Autodesk Inventor part; units mm, degrees
(part 2 of 2)
sketch "Sketch182" plane through (0, 0, 82.74) normal (0, 0, 1) x (1, 0, 0)
  circle A0 centre (-26.5, 130) radius 1.5
  line L0 (-22.5, 136) -> (-22.5, 124) projected
  line L1 (-30.5, 124) -> (-30.5, 136) projected
  line L2 (-22.5, 124) -> (-30.5, 124) projected
  line L3 (-30.5, 136) -> (-22.5, 136) projected
  point P0 (0, 0)
  dimension "d607" = 8
  dimension "d608" = 4
  dimension "d609" = 12
  dimension "d610" = 6
  dimension "d611" = 3
  constraints: 1 centre point
  measures "d607" distance between parallel lines of L0 L1
  measures "d608" distance from line of L0 A0.centre
  measures "d609" distance between parallel lines of L2 L3
  measures "d610" distance from line of L3 A0.centre
  measures "d611" diameter of A0
extrude "Extrusion120" cut sketch "Sketch182" against normal blind 6 contours A0
ref_plane "Work Plane22" through (0, 0, 77) normal (0, 0, 1) x (1, 0, 0)
sketch "Sketch192" plane through (0, 55, 150) normal (0, 1, 0) x (1, 0, 0)
  line L0 (62, 25) -> (57, 25)
  line L1 (57, 25) -> (57, 30)
  line L2 (57, 30) -> (62, 30)
  line L3 (62, 30) -> (62, 25)
  line L4 (62, 25) -> (12, 25) projected
  line L5 (62, 75) -> (62, 25) projected
  line L6 (62, 75) -> (57, 75)
  line L7 (57, 75) -> (57, 70)
  line L8 (57, 70) -> (62, 70)
  line L9 (62, 70) -> (62, 75)
  line L10 (12, 25) -> (17, 25)
  line L11 (17, 25) -> (17, 30)
  line L12 (17, 30) -> (12, 30)
  line L13 (12, 30) -> (12, 25)
  line L14 (12, 75) -> (17, 75)
  line L15 (17, 75) -> (17, 70)
  line L16 (17, 70) -> (12, 70)
  line L17 (12, 70) -> (12, 75)
  point P0 (0, 150)
  dimension "d635" = 5
  constraints: 32 end point, 8 parallel, 7 equal length, 4 horizontal, 4 perpendicular, 3 point on line, 1 coincident
  measures "d635" distance of L1.end L2.end
extrude "Extrusion122" add sketch "Sketch192" against normal blind 3
sketch "Sketch193" plane through (-5, -5, 150) normal (0, -1, 0) x (1, 0, 0)
  line L0 (86.0111, 0) -> (16.0111, 0)
  line L1 (16.0111, 0) -> (16.0111, -137.496)
  line L2 (16.0111, -137.496) -> (86.0111, -137.496)
  line L3 (86.0111, -137.496) -> (86.0111, 0)
  line L4 (0, 0) -> (155, 0) projected
  line L5 (76.0111, -37.496) -> (76.0111, -87.496) projected
  line L6 (26.0111, -87.496) -> (26.0111, -37.496) projected
  line L7 (76.0111, -87.496) -> (26.0111, -87.496) projected
  point P0 (5, -150)
  dimension "d638" = 10
  dimension "d639" = 10
  dimension "d640" = 50
  constraints: 8 end point, 2 parallel, 1 horizontal, 1 perpendicular, 1 point on line
  measures "d638" distance between parallel lines of L3 L5
  measures "d639" distance between parallel lines of L1 L6
  measures "d640" distance between parallel lines of L7 L2
extrude "Extrusion123" add sketch "Sketch193" along normal blind 10
sketch "Sketch194" plane through (-5, -15, 150) normal (0, -1, 0) x (1, 0, 0)
  line L0 (76.0111, -37.496) -> (26.0111, -37.496) projected
  line L1 (76.0111, -87.496) -> (76.0111, -37.496) projected
  line L2 (26.0111, -37.496) -> (76.0111, -37.496)
  line L3 (76.0111, -37.496) -> (76.0111, -87.496)
  line L4 (76.0111, -87.496) -> (26.0111, -87.496)
  line L5 (26.0111, -87.496) -> (26.0111, -37.496)
  point P0 (5, -150)
  constraints: 8 end point, 2 parallel, 1 horizontal, 1 perpendicular
extrude "Extrusion124" cut sketch "Sketch194" against normal up to surface (15 mm away)
sketch "Sketch195" plane through (72, 0, 150) normal (0, 1, 0) x (1, 0, 0)
  line L0 (-0.9889, 87.496) -> (-0.9889, 37.496) projected
  line L1 (-0.9889, 37.496) -> (-5.9889, 37.496)
  line L2 (-5.9889, 37.496) -> (-5.9889, 42.496)
  line L3 (-5.9889, 42.496) -> (-0.9889, 42.496)
  line L4 (-0.9889, 42.496) -> (-0.9889, 37.496)
  line L5 (-50.9889, 87.496) -> (-0.9889, 87.496) projected
  line L6 (-0.9889, 87.496) -> (-5.9889, 87.496)
  line L7 (-5.9889, 87.496) -> (-5.9889, 82.496)
  line L8 (-5.9889, 82.496) -> (-0.9889, 82.496)
  line L9 (-0.9889, 82.496) -> (-0.9889, 87.496)
  line L10 (-50.9889, 37.496) -> (-50.9889, 87.496) projected
  line L11 (-50.9889, 87.496) -> (-45.9889, 87.496)
  line L12 (-45.9889, 87.496) -> (-45.9889, 82.496)
  line L13 (-45.9889, 82.496) -> (-50.9889, 82.496)
  line L14 (-50.9889, 82.496) -> (-50.9889, 87.496)
  line L15 (-0.9889, 37.496) -> (-50.9889, 37.496) projected
  line L16 (-50.9889, 37.496) -> (-45.9889, 37.496)
  line L17 (-45.9889, 37.496) -> (-45.9889, 42.496)
  line L18 (-45.9889, 42.496) -> (-50.9889, 42.496)
  line L19 (-50.9889, 42.496) -> (-50.9889, 37.496)
  point P0 (-72, 150)
  point P1 (-0.9889, 82.496)
  dimension "d645" = 5
  constraints: 32 end point, 8 parallel, 7 equal length, 4 horizontal, 4 perpendicular
  measures "d645" distance of L16.end L17.end
extrude "Extrusion125" add sketch "Sketch195" against normal blind 3 contours L0 L8 L7 L5 | L0 L1 L2 L3 | L12 L13 L10 L5 | L15 L10 L18 L17
sketch "Sketch196" plane through (-65, 65, 150) normal (0, -1, 0) x (1, 0, 0)
  line L0 (12, -83.999) -> (9, -83.999)
  line L1 (9, -83.999) -> (9, -153)
  line L2 (9, -153) -> (12, -153)
  line L3 (12, -153) -> (12, -83.999)
  line L4 (5, -86.999) -> (5, -175) projected
  line L5 (0, -86.999) -> (5, -86.999) projected
  line L6 (170, -150) -> (190, -150) projected
  line L7 (190, -150) -> (170, -150) projected
  line L8 (210, -150) -> (190, -150) projected
  line L9 (190, -150) -> (95, -150) projected
  line L10 (95, -150) -> (142, -150) projected
  line L11 (142, -150) -> (190, -150) projected
  line L12 (190, -150) -> (210, -150) projected
  line L13 (132.0208, -150) -> (128.4853, -150) projected
  line L14 (128.4853, -150) -> (107.9792, -150) projected
  line L15 (107.9792, -150) -> (111.5147, -150) projected
  line L16 (111.5147, -150) -> (132.0208, -150) projected
  line L17 (150, -150) -> (160, -150) projected
  line L18 (160, -150) -> (150, -150) projected
  line L19 (65, -155) -> (210, -155) projected
  line L20 (65, -155) -> (210, -155) projected
  line L21 (65, -155) -> (210, -155) projected
  point P0 (65, -150)
  point P1 (5, -150)
  dimension "d648" = 4
  dimension "d649" = 3
  dimension "d650" = 3
  dimension "d651" = 5
  dimension "d652" = 3
  constraints: 8 end point, 2 parallel, 1 horizontal, 1 perpendicular
  measures "d648" distance between parallel lines of L4 L1
  measures "d649" distance from line of point (5, -150) L2
  measures "d650" distance between parallel lines of L0 L5
  measures "d651" distance from line of L21 point (5, -150)
  measures "d652" distance between parallel lines of L1 L3
extrude "Extrusion126" cut sketch "Sketch196" against normal up to surface (120 mm away)
sketch "Sketch197" plane through (-60, 65, -5) normal (-1, 0, 0) x (0, 0, 1)
  line L0 (-18, 117) -> (3, 117)
  line L1 (3, 117) -> (3, 114)
  line L2 (3, 114) -> (-18, 114)
  line L3 (-18, 114) -> (-18, 117)
  line L4 (68.001, 120) -> (-20, 120) projected
  line L5 (-15, 120) -> (-15, 3) projected
  line L6 (0, 120) -> (0, 3) projected
  point P0 (5, -65)
  dimension "d655" = 3
  dimension "d656" = 3
  dimension "d657" = 3
  dimension "d658" = 3
  constraints: 8 end point, 2 parallel, 1 horizontal, 1 perpendicular
  measures "d655" distance between parallel lines of L4 L0
  measures "d656" distance of L0.end L1.end
  measures "d657" distance between parallel lines of L5 L3
  measures "d658" distance between parallel lines of L6 L1
extrude "Extrusion127" cut sketch "Sketch197" against normal up to surface (210 mm away) contours L0 L5 L2 L3 | L0 L6 L2 L5 | L0 L1 L2 L6
sketch "Sketch198" plane through (-5, -5, 150) normal (-1, 0, 0) x (0, 0, 1)
  line L0 (-173, 6) -> (-152, 6)
  line L1 (-152, 6) -> (-152, 3)
  line L2 (-152, 3) -> (-173, 3)
  line L3 (-173, 3) -> (-173, 6)
  line L4 (-175, 0) -> (0, 0) projected
  point P0 (-150, 5)
  point P1 (-155, 0)
  point P2 (-170, 0)
  dimension "d661" = 3
  dimension "d662" = 3
  dimension "d663" = 3
  dimension "d664" = 3
  constraints: 8 end point, 2 parallel, 1 horizontal, 1 perpendicular
  measures "d661" distance between parallel lines of L4 L2
  measures "d662" distance between parallel lines of L0 L2
  measures "d663" distance from line of point (-155, 0) L1
  measures "d664" distance from line of L3 point (-170, 0)
extrude "Extrusion128" cut sketch "Sketch198" against normal up to surface (155 mm away)
sketch "Sketch203" plane through (0, 0, 150) normal (0, 0, 1) x (1, 0, 0)
  line L0 (60, 28.3) -> (50, 28.3) projected
  line L1 (48.4237, 33.6572) -> (60, 33.6572)
  line L2 (60, 33.6572) -> (60, 28.3)
  line L3 (60, 28.3) -> (48.4237, 28.3)
  line L4 (48.4237, 28.3) -> (48.4237, 33.6572)
  point P0 (0, 0)
  point P1 (53, 28.3)
  point P2 (57, 28.3)
  constraints: 8 end point, 2 parallel, 1 horizontal, 1 perpendicular
extrude "Extrusion129" cut sketch "Sketch203" against normal up to surface (150 mm away)
sketch "Sketch205" plane through (0, 0, 67) normal (0, 0, 1) x (1, 0, 0)
  line L0 (0.6988, 151.5) -> (0.6988, 113) projected
  line L1 (-9.9078, 140) -> (-9.9078, 113) projected
  line L2 (-22.5, 124) -> (-30.5, 124) projected
  line L3 (-30.5, 136) -> (-22.5, 136) projected
  circle A0 centre (-4.6012, 130) radius 15.5
  circle A1 centre (-4.6012, 130) radius 17.2238
  point P0 (0, 0)
  dimension "d678" = 10.6066
  dimension "d679" = 12
  dimension "d680" = 31
  dimension "d681" = 6
  dimension "d683" = 5.3
  constraints: 2 centre point, 1 coincident
  measures "d678" distance between parallel lines of L0 L1
  measures "d679" distance between parallel lines of L2 L3
  measures "d680" diameter of A0
  measures "d681" distance from line of L3 A0.centre
  measures "d683" distance from line of L0 A0.centre
extrude "Extrusion130" add sketch "Sketch205" along normal blind 10 contours A1 L0 A0 | L0 A0 L1 A1 | L1 A0 L0 A1
sketch "Sketch206" plane through (0, 0, 67) normal (0, 0, 1) x (1, 0, 0)
  circle A0 centre (-4.6012, 130) radius 8.89
  arc A1 (0.6988, 144.5657) -> (-9.9078, 144.5633) centre (-4.6012, 130) ccw projected
  point P0 (0, 0)
  point P1 (5.2095, 118)
  point P2 (-14.4119, 118)
  dimension "d686" = 17.78
  constraints: 1 centre point, 1 concentric
  measures "d686" diameter of A0
extrude "Extrusion131" cut sketch "Sketch206" against normal up to surface (4 mm away)
sketch "Sketch207" plane through (0.6988, 140, 67) normal (-1, 0, 0) x (0, 0, 1)
  line L0 (31.7021, 6.386) -> (31.7021, 0)
  line L1 (31.7021, 0) -> (0, 0)
  line L2 (0, 0) -> (0, 4.5657) projected
  line L3 (0, 0) -> (0, 4.8278)
  line L4 (0, 4.8278) -> (10, 4.8278)
  line L5 (10, 6.386) -> (10, 7.2238) projected
  line L6 (10, 4.8278) -> (10, 6.386)
  line L7 (10, 6.386) -> (31.7021, 6.386)
  line L8 (0, 0) -> (36.0104, 0) projected
  point P0 (-67, -140)
  point P1 (10, 6.3881)
  constraints: 12 end point, 3 perpendicular, 2 point on line, 2 vertical, 1 parallel
extrude "Extrusion132" cut sketch "Sketch207" against normal blind 10
sketch "Sketch208" plane through (-8.14, 140, 67) normal (1, 0, 0) x (0, 0, -1)
  line L0 (0, 4) -> (0, 0) projected
  line L1 (0, 0) -> (-23.1716, 0) projected
  line L2 (0, 4) -> (-16.0959, 4)
  line L3 (-16.0959, 4) -> (-16.0959, 0)
  line L4 (-16.0959, 0) -> (0, 0)
  line L5 (0, 0) -> (0, 4)
  point P0 (67, -140)
  constraints: 8 end point, 2 parallel, 1 horizontal, 1 perpendicular, 1 point on line
extrude "Extrusion133" cut sketch "Sketch208" against normal blind 10
sketch "Sketch209" plane through (0, 0, 150) normal (0, 0, 1) x (1, 0, 0)
  line L0 (11.0111, -5) -> (11.0111, -15) projected
  line L1 (81.0111, -5) -> (81.0111, -15) projected
  line L2 (11.0111, -15) -> (81.0111, -15)
  line L3 (81.0111, -15) -> (81.0111, -10)
  line L4 (81.0111, -10) -> (11.0111, -10)
  line L5 (11.0111, -10) -> (11.0111, -15)
  point P0 (0, 0)
  dimension "d693" = 5
  dimension "d694" = 70
  constraints: 8 end point, 2 parallel, 1 horizontal, 1 midpoint, 1 perpendicular
  measures "d693" distance between parallel lines of L2 L4
  measures "d694" distance of L3.end L4.end
extrude "Extrusion134" cut sketch "Sketch209" against normal up to surface (137.496 mm away)
sketch "Sketch210" plane through (0, 0, 150) normal (0, 0, 1) x (1, 0, 0)
  line L0 (0, 27) -> (72, 27) projected
  line L1 (47.5453, 27) -> (62.1225, 27)
  line L2 (62.1225, 27) -> (62.1225, 32.383)
  line L3 (62.1225, 32.383) -> (47.5453, 32.383)
  line L4 (47.5453, 32.383) -> (47.5453, 27)
  point P0 (0, 0)
  constraints: 8 end point, 2 parallel, 1 horizontal, 1 perpendicular, 1 point on line
extrude "Extrusion135" cut sketch "Sketch210" against normal up to surface (150 mm away)
sketch "Sketch211" plane through (-9.9078, 151.5, 92.4038) normal (1, 0, 0) x (0, 0, -1)
  line L0 (25.4038, -6.9367) -> (25.4038, -7.5) projected
  line L1 (25.4038, -6.9367) -> (15.4038, -6.9367) projected
  line L2 (25.4038, -7.5) -> (15.4038, -7.5)
  line L3 (15.4038, -7.5) -> (15.4038, -6.9367)
  line L4 (15.4038, -6.9367) -> (25.4038, -6.9367)
  line L5 (25.4038, -6.9367) -> (25.4038, -7.5)
  point P0 (92.4038, -151.5)
  constraints: 8 end point, 2 parallel, 1 horizontal, 1 perpendicular
extrude "Extrusion136" cut sketch "Sketch211" against normal blind 25.4
thread "Thread9" size "5-40 UNC" class "2B" standard "ANSI Unified Screw Threads" full length
sketch "Sketch212" plane through (-35, 70, 150) normal (1, 0, 0) x (0, 0, -1)
  circle A0 centre (50, 60) radius 10 projected
  line L0 (83, 20) -> (83, 90) projected
  line L1 (150, 110) -> (150, 0) projected
  point P0 (150, -70)
  dimension "d703" = 33
  dimension "d704" = 100
  measures "d703" distance from line of L0 A0.centre
  measures "d704" distance from line of L1 A0.centre
ref_plane "Work Plane24" through (145, 62, -5) normal (0, 0, -1) x (-1, 0, 0)
sketch "Sketch213" plane through (-65, 65, 150) normal (-1, 0, 0) x (0, 0, 1)
  line L0 (-87, 115) -> (-150, 115) projected
  line L1 (-86.999, 120) -> (-86.999, 0) projected
  line L2 (-150, 5) -> (-150, 115) projected
  line L3 (-87, 5) -> (-150, 5) projected
  line L4 (-173, 117) -> (-152, 117) projected
  line L5 (-152, 114) -> (-173, 114) projected
  line L6 (-152, 117) -> (-152, 114) projected
  line L7 (-173, 114) -> (-173, 117) projected
  line L8 (-86.999, 120) -> (-175, 120) projected
  line L9 (-86.999, 120) -> (-175, 120)
  line L10 (-175, 120) -> (-175, 0)
  line L11 (-175, 0) -> (-86.999, 0)
  line L12 (-86.999, 0) -> (-86.999, 120)
  point P0 (-150, -65)
  point P1 (-86.999, 0)
  constraints: 8 end point, 2 parallel, 1 horizontal, 1 perpendicular
ref_plane "Work Plane25" through (-90.4, 65, 150) normal (-1, 0, 0) x (0, 0, 1)
sketch "Sketch214" plane through (-90.4, 65, 150) normal (-1, 0, 0) x (0, 0, 1)
  line L0 (-173, 117) -> (-152, 117) projected
  line L1 (-152, 114) -> (-173, 114) projected
  line L2 (-152, 117) -> (-152, 114) projected
  line L3 (-173, 114) -> (-173, 117) projected
  line L4 (-87, 115) -> (-150, 115) projected
  line L5 (-150, 5) -> (-150, 115) projected
  line L6 (-87, 8) -> (-150, 8) projected
  line L7 (-150, 5) -> (-87, 5) projected
  line L8 (-86.999, 0) -> (-86.999, 120) projected
  point P0 (-150, -65)
extrude "Extrusion137" add sketch "Sketch213" against normal up to surface (5 mm away)
sketch "Sketch215" plane through (-65, 65, 150) normal (-1, 0, 0) x (0, 0, 1)
  line L0 (-150, 115) -> (-87, 115) projected
  line L1 (-87, 115) -> (-150, 115)
  line L2 (-150, 115) -> (-150, 5.0928)
  line L3 (-150, 5.0928) -> (-87, 5.0928)
  line L4 (-87, 5.0928) -> (-87, 115)
  point P0 (-150, -65)
  constraints: 8 end point, 2 parallel, 1 horizontal, 1 perpendicular
extrude "Extrusion138" cut sketch "Sketch215" against normal up to surface (12 mm away)
split body "Split1" result two bodies by plane through (145, 62, -5) normal (0, 0, -1) first body at (98.3333, 81.6667, -24.5)
body "Solid2"
body "Solid3"
